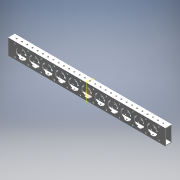
# Autodesk Inventor part: Front Extrusion
Saved by Autodesk Inventor 2019.4 (Build 234330000, 330)
## iProperties
Created: 2019-12-11
Part Number: Front Extrusion
Material: Aluminum 6061
Document SubType Name: Modeling
Designer: Mark
Mass: 882.774 g
Surface Area: 2224.42 cm^2
Volume: 326.953 cm^3
Density: 2.7 g/cm^3
Appearance: Aluminum - Flat
Author: Mark
Autodesk Inventor part; units mm, degrees
ref_plane "YZ Plane" through (0, 0, 0) normal (1, 0, 0) x (0, 1, 0)
ref_plane "XZ Plane" through (0, 0, 0) normal (0, 1, 0) x (-1, 0, 0)
ref_plane "XY Plane" through (0, 0, 0) normal (0, 0, 1) x (1, 0, 0)
sketch "Sketch1" plane through (0, 0, 0) normal (1, 0, 0) x (0, 1, 0)
  line L0 (-30, 12.5) -> (30, 12.5)
  line L1 (30, 12.5) -> (30, -12.5)
  line L2 (30, -12.5) -> (-30, -12.5)
  line L3 (-30, -12.5) -> (-30, 12.5)
  line L4 (-30, 12.5) -> (30, -12.5) construction
  line L5 (30, 12.5) -> (-30, -12.5) construction
  line L6 (-27, 9.5) -> (27, 9.5)
  line L7 (27, 9.5) -> (27, -9.5)
  line L8 (27, -9.5) -> (-27, -9.5)
  line L9 (-27, -9.5) -> (-27, 9.5)
  line L10 (-27, 9.5) -> (27, -9.5) construction
  line L11 (27, 9.5) -> (-27, -9.5) construction
  point P0 (0, 0)
  dimension "d0" = 60
  dimension "d1" = 25
  dimension "d2" = 54
  dimension "d3" = 19
  constraints: 24 end point, 4 midpoint, 4 parallel, 2 horizontal, 2 perpendicular
  measures "d0" distance of L1.end L2.end
  measures "d1" distance of L0.end L1.end
  measures "d2" distance of L7.end L8.end
  measures "d3" distance of L6.end L7.end
extrude "Extrusion1" add sketch "Sketch1" along normal blind 600
ref_plane "Work Plane1" through (300, 0, 0) normal (1, 0, 0) x (0, 0, -1)
sketch "Sketch2" plane through (0, 30, 12.5) normal (0, 1, 0) x (1, 0, 0)
  circle A0 centre (20, 12.5) radius 2.75
  line L0 (0, 0) -> (0, 25) projected
  line L1 (0, 0) -> (600, 0) projected
  circle A1 centre (40, 12.5) radius 2.75
  circle A2 centre (60, 12.5) radius 2.75
  circle A3 centre (80, 12.5) radius 2.75
  circle A4 centre (100, 12.5) radius 2.75
  circle A5 centre (120, 12.5) radius 2.75
  circle A6 centre (140, 12.5) radius 2.75
  circle A7 centre (160, 12.5) radius 2.75
  circle A8 centre (180, 12.5) radius 2.75
  circle A9 centre (200, 12.5) radius 2.75
  circle A10 centre (220, 12.5) radius 2.75
  circle A11 centre (240, 12.5) radius 2.75
  circle A12 centre (260, 12.5) radius 2.75
  circle A13 centre (280, 12.5) radius 2.75
  circle A14 centre (300, 12.5) radius 2.75
  circle A15 centre (320, 12.5) radius 2.75
  circle A16 centre (340, 12.5) radius 2.75
  circle A17 centre (360, 12.5) radius 2.75
  circle A18 centre (380, 12.5) radius 2.75
  circle A19 centre (400, 12.5) radius 2.75
  circle A20 centre (420, 12.5) radius 2.75
  circle A21 centre (440, 12.5) radius 2.75
  circle A22 centre (460, 12.5) radius 2.75
  circle A23 centre (480, 12.5) radius 2.75
  circle A24 centre (500, 12.5) radius 2.75
  circle A25 centre (520, 12.5) radius 2.75
  circle A26 centre (540, 12.5) radius 2.75
  circle A27 centre (560, 12.5) radius 2.75
  circle A28 centre (580, 12.5) radius 2.75
  circle A29 centre (600, 12.5) radius 2.75
  circle A30 centre (620, 12.5) radius 2.75
  circle A31 centre (640, 12.5) radius 2.75
  circle A32 centre (660, 12.5) radius 2.75
  circle A33 centre (680, 12.5) radius 2.75
  circle A34 centre (700, 12.5) radius 2.75
  circle A35 centre (720, 12.5) radius 2.75
  circle A36 centre (740, 12.5) radius 2.75
  circle A37 centre (760, 12.5) radius 2.75
  circle A38 centre (780, 12.5) radius 2.75
  circle A39 centre (800, 12.5) radius 2.75
  circle A40 centre (820, 12.5) radius 2.75
  circle A41 centre (840, 12.5) radius 2.75
  circle A42 centre (860, 12.5) radius 2.75
  circle A43 centre (880, 12.5) radius 2.75
  circle A44 centre (900, 12.5) radius 2.75
  circle A45 centre (920, 12.5) radius 2.75
  circle A46 centre (940, 12.5) radius 2.75
  circle A47 centre (960, 12.5) radius 2.75
  circle A48 centre (980, 12.5) radius 2.75
  circle A49 centre (1000, 12.5) radius 2.75
  point P0 (0, 12.5)
  dimension "d7" = 5.5
  dimension "d8" = 20
  dimension "d9" = 12.5
  dimension "d12" = 20
  constraints: 50 centre point, 1 horizontal, 98 other
  measures "d7" diameter of A0
  measures "d8" distance from line of A0.centre L0
  measures "d9" distance from line of L1 A0.centre
  measures "d12" distance of A0.centre A1.centre
extrude "Extrusion2" cut sketch "Sketch2" against normal blind 100 contours A0 | A1 | A2 | A3 | A4 | A5 | A6 | A7 | A8 | A9 | A10 | A11 | A12 | A13 | A14 | A15 | A16 | A17 | A18 | A19 | A20 | A21 | A22 | A23 | A24 | A25 | A26 | A27 | A28
sketch "Sketch4" plane through (0, -30, 12.5) normal (0, 0, 1) x (1, 0, 0)
  circle A0 centre (300, 30) radius 20
  line L0 (600, 60) -> (600, 0) projected
  line L1 (0, 60) -> (600, 60) projected
  line L2 (275, 7.5) -> (325, 7.5) construction
  line L3 (325, 7.5) -> (325, 52.5) construction
  line L4 (325, 52.5) -> (275, 52.5) construction
  line L5 (275, 52.5) -> (275, 7.5) construction
  line L6 (275, 7.5) -> (325, 52.5) construction
  line L7 (325, 7.5) -> (275, 52.5) construction
  circle A1 centre (275, 52.5) radius 2.75
  circle A2 centre (325, 52.5) radius 2.75
  circle A3 centre (275, 7.5) radius 2.75
  circle A4 centre (325, 7.5) radius 2.5
  circle A5 centre (325, 7.5) radius 2.75
  circle A6 centre (375, 7.5) radius 2.5
  circle A7 centre (375, 52.5) radius 2.75
  circle A8 centre (325, 52.5) radius 2.75
  circle A9 centre (350, 30) radius 20
  circle A10 centre (375, 7.5) radius 2.75
  circle A11 centre (425, 7.5) radius 2.5
  circle A12 centre (425, 52.5) radius 2.75
  circle A13 centre (375, 52.5) radius 2.75
  circle A14 centre (400, 30) radius 20
  circle A15 centre (425, 7.5) radius 2.75
  circle A16 centre (475, 7.5) radius 2.5
  circle A17 centre (475, 52.5) radius 2.75
  circle A18 centre (425, 52.5) radius 2.75
  circle A19 centre (450, 30) radius 20
  circle A20 centre (475, 7.5) radius 2.75
  circle A21 centre (525, 7.5) radius 2.5
  circle A22 centre (525, 52.5) radius 2.75
  circle A23 centre (475, 52.5) radius 2.75
  circle A24 centre (500, 30) radius 20
  circle A25 centre (525, 7.5) radius 2.75
  circle A26 centre (575, 7.5) radius 2.5
  circle A27 centre (575, 52.5) radius 2.75
  circle A28 centre (525, 52.5) radius 2.75
  circle A29 centre (550, 30) radius 20
  circle A30 centre (575, 7.5) radius 2.75
  circle A31 centre (625, 7.5) radius 2.5
  circle A32 centre (625, 52.5) radius 2.75
  circle A33 centre (575, 52.5) radius 2.75
  circle A34 centre (600, 30) radius 20
  circle A35 centre (625, 7.5) radius 2.75
  circle A36 centre (675, 7.5) radius 2.5
  circle A37 centre (675, 52.5) radius 2.75
  circle A38 centre (625, 52.5) radius 2.75
  circle A39 centre (650, 30) radius 20
  circle A40 centre (675, 7.5) radius 2.75
  circle A41 centre (725, 7.5) radius 2.5
  circle A42 centre (725, 52.5) radius 2.75
  circle A43 centre (675, 52.5) radius 2.75
  circle A44 centre (700, 30) radius 20
  circle A45 centre (725, 7.5) radius 2.75
  circle A46 centre (775, 7.5) radius 2.5
  circle A47 centre (775, 52.5) radius 2.75
  circle A48 centre (725, 52.5) radius 2.75
  circle A49 centre (750, 30) radius 20
  circle A50 centre (275, 52.5) radius 2.75
  circle A51 centre (275, 52.5) radius 2.75
  line L8 (275, 7.5) -> (275, 52.5) construction
  circle A52 centre (275, 7.5) radius 2.5
  circle A53 centre (275, 7.5) radius 2.75
  circle A54 centre (250, 30) radius 20
  line L9 (275, 52.5) -> (225, 52.5) construction
  line L10 (225, 7.5) -> (275, 7.5) construction
  line L11 (275, 7.5) -> (225, 52.5) construction
  line L12 (225, 52.5) -> (225, 7.5) construction
  circle A55 centre (225, 52.5) radius 2.75
  circle A56 centre (225, 7.5) radius 2.75
  line L13 (225, 7.5) -> (275, 52.5) construction
  circle A57 centre (225, 52.5) radius 2.75
  circle A58 centre (225, 52.5) radius 2.75
  line L14 (225, 7.5) -> (225, 52.5) construction
  circle A59 centre (225, 7.5) radius 2.5
  circle A60 centre (225, 7.5) radius 2.75
  circle A61 centre (200, 30) radius 20
  line L15 (225, 52.5) -> (175, 52.5) construction
  line L16 (175, 7.5) -> (225, 7.5) construction
  line L17 (225, 7.5) -> (175, 52.5) construction
  line L18 (175, 52.5) -> (175, 7.5) construction
  circle A62 centre (175, 52.5) radius 2.75
  circle A63 centre (175, 7.5) radius 2.75
  line L19 (175, 7.5) -> (225, 52.5) construction
  circle A64 centre (175, 52.5) radius 2.75
  circle A65 centre (175, 52.5) radius 2.75
  line L20 (175, 7.5) -> (175, 52.5) construction
  circle A66 centre (175, 7.5) radius 2.5
  circle A67 centre (175, 7.5) radius 2.75
  circle A68 centre (150, 30) radius 20
  line L21 (175, 52.5) -> (125, 52.5) construction
  line L22 (125, 7.5) -> (175, 7.5) construction
  line L23 (175, 7.5) -> (125, 52.5) construction
  line L24 (125, 52.5) -> (125, 7.5) construction
  circle A69 centre (125, 52.5) radius 2.75
  circle A70 centre (125, 7.5) radius 2.75
  line L25 (125, 7.5) -> (175, 52.5) construction
  circle A71 centre (125, 52.5) radius 2.75
  circle A72 centre (125, 52.5) radius 2.75
  line L26 (125, 7.5) -> (125, 52.5) construction
  circle A73 centre (125, 7.5) radius 2.5
  circle A74 centre (125, 7.5) radius 2.75
  circle A75 centre (100, 30) radius 20
  line L27 (125, 52.5) -> (75, 52.5) construction
  line L28 (75, 7.5) -> (125, 7.5) construction
  line L29 (125, 7.5) -> (75, 52.5) construction
  line L30 (75, 52.5) -> (75, 7.5) construction
  circle A76 centre (75, 52.5) radius 2.75
  circle A77 centre (75, 7.5) radius 2.75
  line L31 (75, 7.5) -> (125, 52.5) construction
  circle A78 centre (75, 52.5) radius 2.75
  circle A79 centre (75, 52.5) radius 2.75
  line L32 (75, 7.5) -> (75, 52.5) construction
  circle A80 centre (75, 7.5) radius 2.5
  circle A81 centre (75, 7.5) radius 2.75
  circle A82 centre (50, 30) radius 20
  line L33 (75, 52.5) -> (25, 52.5) construction
  line L34 (25, 7.5) -> (75, 7.5) construction
  line L35 (75, 7.5) -> (25, 52.5) construction
  line L36 (25, 52.5) -> (25, 7.5) construction
  circle A83 centre (25, 52.5) radius 2.75
  circle A84 centre (25, 7.5) radius 2.75
  line L37 (25, 7.5) -> (75, 52.5) construction
  circle A85 centre (25, 52.5) radius 2.75
  circle A86 centre (25, 52.5) radius 2.75
  line L38 (25, 7.5) -> (25, 52.5) construction
  circle A87 centre (25, 7.5) radius 2.5
  circle A88 centre (25, 7.5) radius 2.75
  circle A89 centre (0, 30) radius 20
  line L39 (25, 52.5) -> (-25, 52.5) construction
  line L40 (-25, 7.5) -> (25, 7.5) construction
  line L41 (25, 7.5) -> (-25, 52.5) construction
  line L42 (-25, 52.5) -> (-25, 7.5) construction
  circle A90 centre (-25, 52.5) radius 2.75
  circle A91 centre (-25, 7.5) radius 2.75
  line L43 (-25, 7.5) -> (25, 52.5) construction
  circle A92 centre (-25, 52.5) radius 2.75
  circle A93 centre (-25, 52.5) radius 2.75
  line L44 (-25, 7.5) -> (-25, 52.5) construction
  circle A94 centre (-25, 7.5) radius 2.5
  circle A95 centre (-25, 7.5) radius 2.75
  circle A96 centre (-50, 30) radius 20
  line L45 (-25, 52.5) -> (-75, 52.5) construction
  line L46 (-75, 7.5) -> (-25, 7.5) construction
  line L47 (-25, 7.5) -> (-75, 52.5) construction
  line L48 (-75, 52.5) -> (-75, 7.5) construction
  circle A97 centre (-75, 52.5) radius 2.75
  circle A98 centre (-75, 7.5) radius 2.75
  line L49 (-75, 7.5) -> (-25, 52.5) construction
  circle A99 centre (-75, 52.5) radius 2.75
  circle A100 centre (-75, 52.5) radius 2.75
  line L50 (-75, 7.5) -> (-75, 52.5) construction
  circle A101 centre (-75, 7.5) radius 2.5
  circle A102 centre (-75, 7.5) radius 2.75
  circle A103 centre (-100, 30) radius 20
  line L51 (-75, 52.5) -> (-125, 52.5) construction
  line L52 (-125, 7.5) -> (-75, 7.5) construction
  line L53 (-75, 7.5) -> (-125, 52.5) construction
  line L54 (-125, 52.5) -> (-125, 7.5) construction
  circle A104 centre (-125, 52.5) radius 2.75
  circle A105 centre (-125, 7.5) radius 2.75
  line L55 (-125, 7.5) -> (-75, 52.5) construction
  circle A106 centre (-125, 52.5) radius 2.75
  circle A107 centre (-125, 52.5) radius 2.75
  line L56 (-125, 7.5) -> (-125, 52.5) construction
  circle A108 centre (-125, 7.5) radius 2.5
  circle A109 centre (-125, 7.5) radius 2.75
  circle A110 centre (-150, 30) radius 20
  line L57 (-125, 52.5) -> (-175, 52.5) construction
  line L58 (-175, 7.5) -> (-125, 7.5) construction
  line L59 (-125, 7.5) -> (-175, 52.5) construction
  line L60 (-175, 52.5) -> (-175, 7.5) construction
  circle A111 centre (-175, 52.5) radius 2.75
  circle A112 centre (-175, 7.5) radius 2.75
  line L61 (-175, 7.5) -> (-125, 52.5) construction
  dimension "d34" = 40
  dimension "d35" = 300
  dimension "d36" = 30
  dimension "d37" = 50
  dimension "d38" = 45
  dimension "d39" = 5.5
  dimension "d40" = 5.5
  dimension "d41" = 5.5
  dimension "d42" = 5
  dimension "d45" = 50
  dimension "d55" = 50
  constraints: 120 end point, 113 centre point, 40 coincident, 20 midpoint, 3 horizontal, 2 parallel, 1 perpendicular, 306 other
  measures "d34" diameter of A0
  measures "d35" distance from line of L0 A0.centre
  measures "d36" distance from line of L1 A0.centre
  measures "d37" distance of L4.end L3.end
  measures "d38" distance of L3.end L2.end
  measures "d39" diameter of A1
  measures "d40" diameter of A2
  measures "d41" diameter of A3
  measures "d42" diameter of A4
  measures "d45" distance of A3.centre A5.centre
  measures "d55" distance of L3.end L8.end
extrude "Extrusion3" cut sketch "Sketch4" against normal blind 30 contours A0 | A1 | A2 | A3 | A4 | A5 | A6 | A7 | A9 | A10 | A11 | A12 | A14 | A15 | A16 | A17 | A19 | A20 | A21 | A22 | A24 | A25 | A26 | A27 | A29 | A52 | A54 | A55 | A56 | A59 | A61 | A62 | A63 | A66 | A68 | A69 | A70 | A73 | A75 | A76 | A77 | A80 | A82 | A83 | A84 | A87
equation "\"d4\" = Width"
equation "\"Width\" = 600"
body "Solid1"
